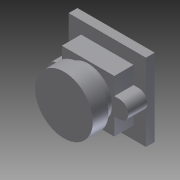
# Autodesk Inventor part: camera
Saved by Autodesk Inventor 2011 (Build 150239000, 239)
## iProperties
Created: 2011-03-05
Part Number: camera
Document SubType Name: Modeling
Designer: labuser
Density: 1 g/cm^3
Author: labuser
Autodesk Inventor part; units mm, degrees
ref_plane "YZ Plane" through (0, 0, 0) normal (1, 0, 0) x (0, 1, 0)
ref_plane "XZ Plane" through (0, 0, 0) normal (0, 1, 0) x (-1, 0, 0)
ref_plane "XY Plane" through (0, 0, 0) normal (0, 0, 1) x (1, 0, 0)
sketch "Sketch1" plane through (0, 0, 0) normal (0, 0, 1) x (1, 0, 0)
  line L0 (0, 0) -> (15, 0) construction
  line L1 (15, 0) -> (15, 15) construction
  line L2 (15, 15) -> (0, 15) construction
  line L3 (0, 15) -> (0, 0) construction
  circle A0 centre (-1.5, 7.5) radius 2.5 construction
  circle A1 centre (16.5, 7.5) radius 2.5 construction
  line L4 (0, 15) -> (15, 15)
  line L5 (0, 0) -> (15, 0)
  arc A2 (-1.5, 10) -> (-1.5, 5) centre (-1.5, 7.5) ccw
  arc A3 (16.5, 5) -> (16.5, 10) centre (16.5, 7.5) ccw
  line L6 (-1.5, 10) -> (0, 10)
  line L7 (-1.5, 5) -> (0, 5)
  line L8 (16.5, 10) -> (15, 10)
  line L9 (16.5, 5) -> (15, 5)
  line L10 (15, 10) -> (15, 15)
  line L11 (0, 10) -> (0, 15)
  line L12 (0, 5) -> (0, 0)
  line L13 (15, 0) -> (15, 5)
  dimension "d0" = 15
  dimension "d1" = 15
  dimension "d2" = 5
  dimension "d3" = 5
  constraints: 28 end point, 10 tangent, 8 point on circle, 6 collinear, 5 perpendicular, 4 centre point, 4 point on line, 2 parallel, 1 horizontal
  measures "d0" distance of L2.end L1.end
  measures "d1" distance of L1.end L0.end
  measures "d2" diameter of A0
  measures "d3" diameter of A1
extrude "Extrusion1" add sketch "Sketch1" along normal blind 5.5
sketch "Sketch2" plane through (0, 0, 5.5) normal (0, 0, 1) x (1, 0, 0)
  line L0 (0, 5) -> (-1.5, 5) projected
  line L1 (7.5, 18.6806) -> (7.5, -6.0082)
  line L2 (-7.546, 7.5) -> (23.0032, 7.5)
  circle A0 centre (7.5, 7.5) radius 6.85
  dimension "d6" = 13.7
  constraints: 4 end point, 2 perpendicular, 2 point on line, 1 centre point
  measures "d6" diameter of A0
extrude "Extrusion2" add sketch "Sketch2" along normal blind 2.4
sketch "Sketch3" plane through (7.5, 7.5, 7.9) normal (0, 0, 1) x (1, 0, 0)
  circle A0 centre (0, 0) radius 6.85 projected
  circle A1 centre (0, 0) radius 8.25
  point P0 (-7.5, -7.5)
  dimension "d9" = 16.5
  constraints: 1 centre point, 1 coincident
  measures "d9" diameter of A1
extrude "Extrusion3" add sketch "Sketch3" along normal blind 4.5 contours A0 | A1
sketch "Sketch4" plane through (0, 0, 0) normal (0, 0, -1) x (-1, 0, 0)
  line L0 (-15, 0) -> (-15, 5) projected
  line L1 (-7.5, 18.462) -> (-7.5, -5.0214)
  line L2 (-22.4523, 7.5) -> (8.5989, 7.5)
  circle A0 centre (-7.5, 7.5) radius 11.05 construction
  line L3 (-18.55, -3.55) -> (3.55, -3.55)
  line L4 (3.55, -3.55) -> (3.55, 18.55)
  line L5 (3.55, 18.55) -> (-18.55, 18.55)
  line L6 (-18.55, 18.55) -> (-18.55, -3.55)
  dimension "d12" = 22.1
  constraints: 12 end point, 3 parallel, 2 perpendicular, 2 point on line, 1 centre point, 1 horizontal
  measures "d12" diameter of A0
extrude "Extrusion4" add sketch "Sketch4" along normal blind 2.5
body "Solid1"
